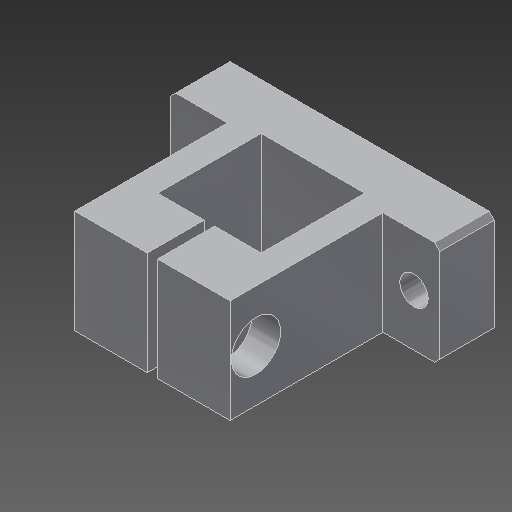
# Autodesk Inventor part: CLTQAM20
Saved by Autodesk Inventor 2021.1 (Build 251245010, 245A)
## iProperties
Created: 2010-03-11
Part Number: CLTQAM20
Material: MISUMI
Document SubType Name: Modeling
Density: 1 g/cm^3
Appearance: アルミニウム - フラット
Title: スタンドブラケット
Autodesk Inventor part; units mm, degrees
note: some values were not read from the file. Chosen so that the rebuilt part matches the saved one: direction of "穴2"; direction of "穴3".
ref_plane "YZ Plane" through (0, 0, 0) normal (1, 0, 0) x (0, 1, 0)
ref_plane "XZ Plane" through (0, 0, 0) normal (0, 1, 0) x (-1, 0, 0)
ref_plane "XY Plane" through (0, 0, 0) normal (0, 0, 1) x (1, 0, 0)
sketch "スケッチ1" plane through (0, 0, 0) normal (0, 0, 1) x (1, 0, 0)
  line L0 (-26, 10) -> (26, 10)
  line L1 (26, 10) -> (26, -10)
  line L2 (26, -10) -> (-26, -10)
  line L3 (-26, -10) -> (-26, 10)
  point P0 (0, 0)
  point P1 (0, -10)
  point P2 (-26, 0)
  dimension "d0" = 52
  dimension "d1" = 20
  constraints: 8 end point, 2 midpoint, 2 parallel, 1 horizontal, 1 horizontal alignment, 1 perpendicular, 1 vertical alignment
  measures "d0" distance of L1.end L2.end
  measures "d1" distance of L2.end L0.start
extrude "押し出し1" add sketch "スケッチ1" along normal blind 10.5
sketch "スケッチ2" plane through (0, 0, 10.5) normal (0, 0, 1) x (1, 0, 0)
  line L0 (-26, 10) -> (26, 10) projected
  line L1 (26, -10) -> (-26, -10) projected
  line L2 (-15, 10) -> (15, 10)
  line L3 (15, 10) -> (15, -10)
  line L4 (15, -10) -> (-15, -10)
  line L5 (-15, -10) -> (-15, 10)
  point P0 (0, 0)
  point P1 (0, -10)
  dimension "d4" = 30
  constraints: 8 end point, 2 parallel, 2 point on line, 1 horizontal, 1 midpoint, 1 perpendicular, 1 vertical alignment
  measures "d4" distance between parallel lines of L3 L5
extrude "押し出し2" add sketch "スケッチ2" along normal blind 29.5
sketch "スケッチ4" plane through (-26, -10, 0) normal (0, -1, 0) x (1, 0, 0)
  line L0 (52, 0) -> (0, 0) projected
  line L1 (16, 29) -> (36, 29)
  line L2 (36, 29) -> (36, 9)
  line L3 (36, 9) -> (16, 9)
  line L4 (16, 9) -> (16, 29)
  point P0 (26, 0)
  point P1 (26, 9)
  point P2 (26, 0)
  dimension "d8" = 20
  dimension "d9" = 20
  dimension "d10" = 9
  constraints: 8 end point, 2 midpoint, 2 parallel, 1 horizontal, 1 perpendicular, 1 vertical alignment
  measures "d8" distance of L2.end L3.end
  measures "d9" distance of L3.end L1.start
  measures "d10" distance between parallel lines of L3 L0
extrude "押し出し3" cut sketch "スケッチ4" against normal through all
sketch "スケッチ5" plane through (0, 0, 40) normal (0, 0, 1) x (1, 0, 0)
  line L0 (-15, 10) -> (15, 10) projected
  line L1 (15, -10) -> (-15, -10) projected
  line L2 (-1, 10) -> (1, 10)
  line L3 (1, 10) -> (1, -10)
  line L4 (1, -10) -> (-1, -10)
  line L5 (-1, -10) -> (-1, 10)
  point P0 (0, 0)
  point P1 (0, -10)
  dimension "d13" = 2
  constraints: 8 end point, 2 parallel, 2 point on line, 1 horizontal, 1 midpoint, 1 perpendicular, 1 vertical alignment
  measures "d13" distance between parallel lines of L5 L3
extrude "押し出し4" cut sketch "スケッチ5" against normal up to surface (11 mm away)
sketch "スケッチ6" plane through (0, 0, 10.5) normal (0, 0, 1) x (1, 0, 0)
  line L0 (-26, -10) -> (-26, 10) projected
  line L1 (26, 10) -> (26, -10) projected
  point P0 (0, 0)
  point P1 (-21, 0)
  point P2 (21, 0)
  point P3 (-26, 0)
  dimension "d16" = 5
  dimension "d17" = 5
  constraints: 2 horizontal alignment, 1 midpoint
  measures "d16" distance from line of point (-21, 0) L0
  measures "d17" distance from line of point (21, 0) L1
hole "穴1" at (-21, 0, 10.5) at (21, 0, 10.5) direction (0, 0, -1) diameter 5.5 end through all
sketch "スケッチ7" plane through (15, -10, 10.5) normal (1, 0, 0) x (0, 0, -1)
  line L0 (-29.5, 20) -> (-29.5, 0) projected
  line L1 (10.5, 12.75) -> (10.5, 7.25) projected
  point P0 (10.5, 10)
  point P1 (-24.5, 10)
  point P2 (-29.5, 10)
  dimension "d25" = 35
  constraints: 1 horizontal alignment, 1 midpoint
  measures "d25" distance from line of L1 point (-24.5, 10)
hole "穴2" at (15, 0, 35) direction (-1, 0, 0) diameter 5.5 end up to surface counterbore diameter 9.5 counterbore depth 5.5
sketch "スケッチ8" plane through (-15, -10, 10.5) normal (-1, 0, 0) x (0, 0, 1)
  circle A0 centre (24.5, 10) radius 2.75 projected
  point P0 (-10.5, 10)
hole "穴3" at (-15, 0, 35) direction (1, 0, 0) diameter 4.134 end up to surface thread size "M5x0.8" class "6H" standard "ANSI Metric M Profile"
chamfer "面取り1" distance 1 angle 45 4 edges at (-26, 10, 5.25) (26, 10, 5.25) (26, -10, 5.25) (-26, -10, 5.25)
equation "\"d9\" = d8"
equation "\"d17\" = d16"
